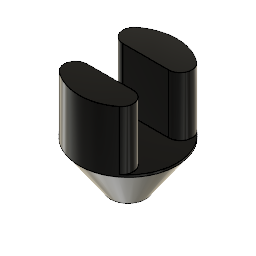
ROV feet v4 (Autodesk Fusion 360 design; units mm, degrees)
Autodesk Fusion 360 part; units mm, degrees
sketch "Sketch1" plane through (0, 0, -115) normal (0, 0, -1) x (1, 0, 0) in component "Component"
  line L0 (138.8604, -9) -> (138.8604, 0)
  line L1 (138.8604, 0) -> (-138.8604, 0)
  line L2 (-138.8604, 0) -> (-138.8604, -9)
  line L3 (-138.8604, -9) -> (138.8604, -9)
  circle A0 centre (95.4863, -4.5) radius 12.5
  dimension "d1" = 25
  measures "d1" diameter of A0
extrude "Extrude1" add sketch "Sketch1" along normal blind 12 contours L3 A0 | L1 L3 A0 | L1 A0 in component "Component"
chamfer "Chamfer1" distance 8 angle 55 1 edges at (83.8322, 9.0202, -127) measured on face at (92.2935, 9.2743, -127) in component "Component"
extrude "Extrude2" add sketch "Sketch1" against normal blind 15 contours L3 A0 | L1 A0 in component "Component"
fillet "Fillet1" radius 3 4 edges at (83.8244, 9, -107.5) (83.8244, 0, -107.5) (107.1482, 0, -107.5) (107.1482, 9, -107.5) in component "Component"
component "Component" placed x (1, 0, 0) y (0, 1, 0) z (0, 0, 1) at (0, 0, 0)
